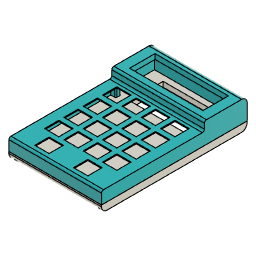
calculator rev1 16122023 (Autodesk Fusion 360 design; units mm, degrees)
Autodesk Fusion 360 part; units mm, degrees
note: some values were not read from the file. Set by a fixed rule: which sketch regions a step uses.
sketch "Sketch1" plane through (0, 0, 0) normal (0, 0, 1) x (1, 0, 0)
  line L0 (-19, 82) -> (72, 82)
  line L1 (72, 82) -> (72, -61)
  line L2 (72, -61) -> (-19, -61)
  line L3 (-19, -61) -> (-19, 82)
  line L4 (-9, 35) -> (5, 35)
  line L5 (5, 35) -> (5, 21)
  line L6 (5, 21) -> (-9, 21)
  line L7 (-9, 21) -> (-9, 35)
  line L8 (10, 35) -> (24, 35)
  line L9 (24, 35) -> (24, 21)
  line L10 (24, 21) -> (10, 21)
  line L11 (10, 21) -> (10, 35)
  line L12 (29, 35) -> (43, 35)
  line L13 (43, 35) -> (43, 21)
  line L14 (43, 21) -> (29, 21)
  line L15 (29, 21) -> (29, 35)
  line L16 (48, 35) -> (62, 35)
  line L17 (62, 35) -> (62, 21)
  line L18 (62, 21) -> (48, 21)
  line L19 (48, 21) -> (48, 35)
  line L20 (-9, 16) -> (5, 16)
  line L21 (5, 16) -> (5, 2)
  line L22 (5, 2) -> (-9, 2)
  line L23 (-9, 2) -> (-9, 16)
  line L24 (10, 16) -> (24, 16)
  line L25 (24, 16) -> (24, 2)
  line L26 (24, 2) -> (10, 2)
  line L27 (10, 2) -> (10, 16)
  line L28 (29, 16) -> (43, 16)
  line L29 (43, 16) -> (43, 2)
  line L30 (43, 2) -> (29, 2)
  line L31 (29, 2) -> (29, 16)
  line L32 (48, 16) -> (62, 16)
  line L33 (62, 16) -> (62, 2)
  line L34 (62, 2) -> (48, 2)
  line L35 (48, 2) -> (48, 16)
  line L36 (-9, -3) -> (5, -3)
  line L37 (5, -3) -> (5, -17)
  line L38 (5, -17) -> (-9, -17)
  line L39 (-9, -17) -> (-9, -3)
  line L40 (10, -3) -> (24, -3)
  line L41 (24, -3) -> (24, -17)
  line L42 (24, -17) -> (10, -17)
  line L43 (10, -17) -> (10, -3)
  line L44 (29, -3) -> (43, -3)
  line L45 (43, -3) -> (43, -17)
  line L46 (43, -17) -> (29, -17)
  line L47 (29, -17) -> (29, -3)
  line L48 (48, -3) -> (62, -3)
  line L49 (62, -3) -> (62, -17)
  line L50 (62, -17) -> (48, -17)
  line L51 (48, -17) -> (48, -3)
  line L52 (-9, -22) -> (5, -22)
  line L53 (5, -22) -> (5, -36)
  line L54 (5, -36) -> (-9, -36)
  line L55 (-9, -36) -> (-9, -22)
  line L56 (10, -22) -> (24, -22)
  line L57 (24, -22) -> (24, -36)
  line L58 (24, -36) -> (10, -36)
  line L59 (10, -36) -> (10, -22)
  line L60 (29, -22) -> (43, -22)
  line L61 (43, -22) -> (43, -36)
  line L62 (43, -36) -> (29, -36)
  line L63 (29, -36) -> (29, -22)
  line L64 (48, -22) -> (62, -22)
  line L65 (62, -22) -> (62, -36)
  line L66 (62, -36) -> (48, -36)
  line L67 (48, -36) -> (48, -22)
  line L68 (0.5, -41) -> (14.5, -41)
  line L69 (14.5, -41) -> (14.5, -55)
  line L70 (14.5, -55) -> (0.5, -55)
  line L71 (0.5, -55) -> (0.5, -41)
  line L72 (38.5, -41) -> (52.5, -41)
  line L73 (52.5, -41) -> (52.5, -55)
  line L74 (52.5, -55) -> (38.5, -55)
  line L75 (38.5, -55) -> (38.5, -41)
  line L76 (-9.5, 73) -> (62.5, 73)
  line L77 (62.5, 73) -> (62.5, 48)
  line L78 (62.5, 48) -> (-9.5, 48)
  line L79 (-9.5, 48) -> (-9.5, 73)
  dimension "d2" = 10
  dimension "d3" = 5
  dimension "d5" = 5
  dimension "d7" = 5
  dimension "d10" = 14
  dimension "d11" = 10
  dimension "d12" = 5
  dimension "d13" = 5
  dimension "d14" = 5
  dimension "d15" = 9.5
  dimension "d16" = 9.5
  dimension "d17" = 14
  dimension "d18" = 5
  dimension "d19" = 5
  dimension "d20" = 25
  dimension "d21" = 72
  dimension "d22" = 91
  dimension "d23" = 9.5
  dimension "d24" = 13
  dimension "d34" = 9
  dimension "d84" = 143
  constraint horizontal L0
  constraint vertical L1
  constraint horizontal L2
  constraint vertical L3
  constraint horizontal L4
  constraint vertical L5
  constraint horizontal L6
  constraint vertical L7
  constraint horizontal L8
  constraint vertical L9
  constraint horizontal L10
  constraint vertical L11
  constraint horizontal L12
  constraint vertical L13
  constraint horizontal L14
  constraint vertical L15
  constraint horizontal L16
  constraint vertical L17
  constraint horizontal L18
  constraint vertical L19
  constraint horizontal L20
  constraint vertical L21
  constraint horizontal L22
  constraint vertical L23
  constraint horizontal L24
  constraint vertical L25
  constraint horizontal L26
  constraint vertical L27
  constraint horizontal L28
  constraint vertical L29
  constraint horizontal L30
  constraint vertical L31
  constraint horizontal L32
  constraint vertical L33
  constraint horizontal L34
  constraint vertical L35
  constraint horizontal L36
  constraint vertical L37
  constraint horizontal L38
  constraint vertical L39
  constraint horizontal L40
  constraint vertical L41
  constraint horizontal L42
  constraint vertical L43
  constraint horizontal L44
  constraint vertical L45
  constraint horizontal L46
  constraint vertical L47
  constraint horizontal L48
  constraint vertical L49
  constraint horizontal L50
  constraint vertical L51
  constraint horizontal L52
  constraint vertical L53
  constraint horizontal L54
  constraint vertical L55
  constraint horizontal L56
  constraint vertical L57
  constraint horizontal L58
  constraint vertical L59
  constraint horizontal L60
  constraint vertical L61
  constraint horizontal L62
  constraint vertical L63
  constraint horizontal L64
  constraint vertical L65
  constraint horizontal L66
  constraint vertical L67
  constraint horizontal L68
  constraint vertical L69
  constraint horizontal L70
  constraint vertical L71
  constraint horizontal L72
  constraint vertical L73
  constraint horizontal L74
  constraint vertical L75
  constraint horizontal L76
  constraint vertical L77
  constraint horizontal L78
  constraint vertical L79
  measures "d2" distance of L3 L7
  measures "d3" distance of L5 L11
  measures "d5" distance of L9 L15
  measures "d7" distance of L13 L19
  measures "d10" distance of L17 L19
  measures "d11" distance of L1 L17
  measures "d12" distance of L6 L20
  measures "d13" distance of L22 L36
  measures "d14" distance of L38 L52
  measures "d15" distance of L57 L69
  measures "d16" distance of L63 L75
  measures "d17" distance of L73 L75
  measures "d18" distance of L58 L68
  measures "d19" distance of L62 L72
  measures "d20" distance of L76 L78
  measures "d21" distance of L77 L79
  measures "d22" distance of L1 L3
  measures "d23" distance of L3 L79
  measures "d24" distance of L4 L78
  measures "d34" distance of L0 L76
  measures "d84" distance of L0 L2
extrude "Extrude1" add sketch "Sketch1" along normal blind 3 makes body 1
sketch "Sketch2" plane through (0, 0, 3) normal (0, 0, 1) x (-1, 0, 0)
  line L0 (-52.5, 55) -> (-38.5, 55)
  line L1 (-38.5, 55) -> (-38.5, 41)
  line L2 (-38.5, 41) -> (-52.5, 41)
  line L3 (-52.5, 41) -> (-52.5, 55)
  line L4 (-62.5, -48) -> (9.5, -48)
  line L5 (9.5, -48) -> (9.5, -73)
  line L6 (9.5, -73) -> (-62.5, -73)
  line L7 (-62.5, -73) -> (-62.5, -48)
  line L8 (-43, -21) -> (-29, -21)
  line L9 (-29, -21) -> (-29, -35)
  line L10 (-29, -35) -> (-43, -35)
  line L11 (-43, -35) -> (-43, -21)
  line L12 (-43, -2) -> (-29, -2)
  line L13 (-29, -2) -> (-29, -16)
  line L14 (-29, -16) -> (-43, -16)
  line L15 (-43, -16) -> (-43, -2)
  line L16 (-24, -2) -> (-10, -2)
  line L17 (-10, -2) -> (-10, -16)
  line L18 (-10, -16) -> (-24, -16)
  line L19 (-24, -16) -> (-24, -2)
  line L20 (-5, -21) -> (9, -21)
  line L21 (9, -21) -> (9, -35)
  line L22 (9, -35) -> (-5, -35)
  line L23 (-5, -35) -> (-5, -21)
  line L24 (-5, -2) -> (9, -2)
  line L25 (9, -2) -> (9, -16)
  line L26 (9, -16) -> (-5, -16)
  line L27 (-5, -16) -> (-5, -2)
  line L28 (-5, 17) -> (9, 17)
  line L29 (9, 17) -> (9, 3)
  line L30 (9, 3) -> (-5, 3)
  line L31 (-5, 3) -> (-5, 17)
  line L32 (-62, -2) -> (-48, -2)
  line L33 (-48, -2) -> (-48, -16)
  line L34 (-48, -16) -> (-62, -16)
  line L35 (-62, -16) -> (-62, -2)
  line L36 (-62, 17) -> (-48, 17)
  line L37 (-48, 17) -> (-48, 3)
  line L38 (-48, 3) -> (-62, 3)
  line L39 (-62, 3) -> (-62, 17)
  line L40 (-43, 17) -> (-29, 17)
  line L41 (-29, 17) -> (-29, 3)
  line L42 (-29, 3) -> (-43, 3)
  line L43 (-43, 3) -> (-43, 17)
  line L44 (-24, 36) -> (-10, 36)
  line L45 (-10, 36) -> (-10, 22)
  line L46 (-10, 22) -> (-24, 22)
  line L47 (-24, 22) -> (-24, 36)
  line L48 (-43, 36) -> (-29, 36)
  line L49 (-29, 36) -> (-29, 22)
  line L50 (-29, 22) -> (-43, 22)
  line L51 (-43, 22) -> (-43, 36)
  line L52 (-62, 36) -> (-48, 36)
  line L53 (-48, 36) -> (-48, 22)
  line L54 (-48, 22) -> (-62, 22)
  line L55 (-62, 22) -> (-62, 36)
  line L56 (-5, 36) -> (9, 36)
  line L57 (9, 36) -> (9, 22)
  line L58 (9, 22) -> (-5, 22)
  line L59 (-5, 22) -> (-5, 36)
  line L60 (-14.5, 55) -> (-0.5, 55)
  line L61 (-0.5, 55) -> (-0.5, 41)
  line L62 (-0.5, 41) -> (-14.5, 41)
  line L63 (-14.5, 41) -> (-14.5, 55)
  line L64 (-24, 17) -> (-10, 17)
  line L65 (-10, 17) -> (-10, 3)
  line L66 (-10, 3) -> (-24, 3)
  line L67 (-24, 3) -> (-24, 17)
  line L68 (-62, -21) -> (-48, -21)
  line L69 (-48, -21) -> (-48, -35)
  line L70 (-48, -35) -> (-62, -35)
  line L71 (-62, -35) -> (-62, -21)
  line L72 (-24, -21) -> (-10, -21)
  line L73 (-10, -21) -> (-10, -35)
  line L74 (-10, -35) -> (-24, -35)
  line L75 (-24, -35) -> (-24, -21)
  line L76 (19, 61) -> (-72, 61)
  line L77 (-72, 61) -> (-72, -82)
  line L78 (-72, -82) -> (19, -82)
  line L79 (19, -82) -> (19, 61)
  line L80 (19, -82) -> (-72, -82)
  line L81 (-72, -82) -> (-72, -43)
  line L82 (-72, -43) -> (19, -43)
  line L83 (19, -43) -> (19, -82)
  dimension "d29" = 5
  constraint horizontal L80
  constraint vertical L81
  constraint horizontal L82
  constraint vertical L83
  constraint coincident L77 L81.end
  constraint coincident L78.end L79.start
  measures "d29" distance of L4 L82
extrude "Extrude2" add sketch "Sketch2" along normal blind 3 contours L77 L78 L79 L80 L81 L82 L83 bodies 1
extrude "Extrude3" add 1 faces at (41.6667, 43, 4) along direction (0, -1, 0) blind 3 on bodies 1 bodies 1
sketch "Sketch3" plane through (0, 0, 0) normal (0, 0, -1) x (1, 0, 0)
  line L0 (-9.5, -48) -> (62.5, -48)
  line L1 (62.5, -48) -> (62.5, -73)
  line L2 (62.5, -73) -> (-9.5, -73)
  line L3 (-9.5, -73) -> (-9.5, -48)
  line L4 (38.5, 55) -> (52.5, 55)
  line L5 (52.5, 55) -> (52.5, 41)
  line L6 (52.5, 41) -> (38.5, 41)
  line L7 (38.5, 41) -> (38.5, 55)
  line L8 (0.5, 55) -> (14.5, 55)
  line L9 (14.5, 55) -> (14.5, 41)
  line L10 (14.5, 41) -> (0.5, 41)
  line L11 (0.5, 41) -> (0.5, 55)
  line L12 (48, 36) -> (62, 36)
  line L13 (62, 36) -> (62, 22)
  line L14 (62, 22) -> (48, 22)
  line L15 (48, 22) -> (48, 36)
  line L16 (29, 36) -> (43, 36)
  line L17 (43, 36) -> (43, 22)
  line L18 (43, 22) -> (29, 22)
  line L19 (29, 22) -> (29, 36)
  line L20 (10, 36) -> (24, 36)
  line L21 (24, 36) -> (24, 22)
  line L22 (24, 22) -> (10, 22)
  line L23 (10, 22) -> (10, 36)
  line L24 (10, 17) -> (24, 17)
  line L25 (24, 17) -> (24, 3)
  line L26 (24, 3) -> (10, 3)
  line L27 (10, 3) -> (10, 17)
  line L28 (29, 17) -> (43, 17)
  line L29 (43, 17) -> (43, 3)
  line L30 (43, 3) -> (29, 3)
  line L31 (29, 3) -> (29, 17)
  line L32 (48, 17) -> (62, 17)
  line L33 (62, 17) -> (62, 3)
  line L34 (62, 3) -> (48, 3)
  line L35 (48, 3) -> (48, 17)
  line L36 (-9, 36) -> (5, 36)
  line L37 (5, 36) -> (5, 22)
  line L38 (5, 22) -> (-9, 22)
  line L39 (-9, 22) -> (-9, 36)
  line L40 (-9, -2) -> (5, -2)
  line L41 (5, -2) -> (5, -16)
  line L42 (5, -16) -> (-9, -16)
  line L43 (-9, -16) -> (-9, -2)
  line L44 (10, -21) -> (24, -21)
  line L45 (24, -21) -> (24, -35)
  line L46 (24, -35) -> (10, -35)
  line L47 (10, -35) -> (10, -21)
  line L48 (29, -21) -> (43, -21)
  line L49 (43, -21) -> (43, -35)
  line L50 (43, -35) -> (29, -35)
  line L51 (29, -35) -> (29, -21)
  line L52 (-9, -21) -> (5, -21)
  line L53 (5, -21) -> (5, -35)
  line L54 (5, -35) -> (-9, -35)
  line L55 (-9, -35) -> (-9, -21)
  line L56 (10, -2) -> (24, -2)
  line L57 (24, -2) -> (24, -16)
  line L58 (24, -16) -> (10, -16)
  line L59 (10, -16) -> (10, -2)
  line L60 (29, -2) -> (43, -2)
  line L61 (43, -2) -> (43, -16)
  line L62 (43, -16) -> (29, -16)
  line L63 (29, -16) -> (29, -2)
  line L64 (48, -2) -> (62, -2)
  line L65 (62, -2) -> (62, -16)
  line L66 (62, -16) -> (48, -16)
  line L67 (48, -16) -> (48, -2)
  line L68 (-9, 17) -> (5, 17)
  line L69 (5, 17) -> (5, 3)
  line L70 (5, 3) -> (-9, 3)
  line L71 (-9, 3) -> (-9, 17)
  line L72 (48, -21) -> (62, -21)
  line L73 (62, -21) -> (62, -35)
  line L74 (62, -35) -> (48, -35)
  line L75 (48, -35) -> (48, -21)
  line L76 (72, 61) -> (-19, 61)
  line L77 (-19, 61) -> (-19, -82)
  line L78 (-19, -82) -> (72, -82)
  line L79 (72, -82) -> (72, 61)
  line L80 (-17, 59) -> (70, 59)
  line L81 (70, 59) -> (70, -80)
  line L82 (70, -80) -> (-17, -80)
  line L83 (-17, -80) -> (-17, 59)
  dimension "d35" = 2
  dimension "d36" = 2
  dimension "d37" = 2
  dimension "d38" = 2
  constraint horizontal L80
  constraint vertical L81
  constraint horizontal L82
  constraint vertical L83
  measures "d35" distance of L79 L81
  measures "d36" distance of L77 L83
  measures "d37" distance of L78 L82
  measures "d38" distance of L76 L80
extrude "Extrude4" cut sketch "Sketch3" against normal blind 2 contours L80 L81 L82 L83 bodies 1
extrude "Extrude5" add 1 faces at (68.8333, 65, 6) along direction (0, 0, 1) blind 10 on bodies 1 bodies 1
sketch "Sketch4" plane through (0, 0, 2) normal (0, 0, -1) x (1, 0, 0)
  line L0 (62, -35) -> (48, -35)
  line L1 (48, -35) -> (48, -21)
  line L2 (48, -21) -> (62, -21)
  line L3 (62, -21) -> (62, -35)
  line L4 (5, 3) -> (-9, 3)
  line L5 (-9, 3) -> (-9, 17)
  line L6 (-9, 17) -> (5, 17)
  line L7 (5, 17) -> (5, 3)
  line L8 (62, -16) -> (48, -16)
  line L9 (48, -16) -> (48, -2)
  line L10 (48, -2) -> (62, -2)
  line L11 (62, -2) -> (62, -16)
  line L12 (43, -16) -> (29, -16)
  line L13 (29, -16) -> (29, -2)
  line L14 (29, -2) -> (43, -2)
  line L15 (43, -2) -> (43, -16)
  line L16 (24, -16) -> (10, -16)
  line L17 (10, -16) -> (10, -2)
  line L18 (10, -2) -> (24, -2)
  line L19 (24, -2) -> (24, -16)
  line L20 (5, -35) -> (-9, -35)
  line L21 (-9, -35) -> (-9, -21)
  line L22 (-9, -21) -> (5, -21)
  line L23 (5, -21) -> (5, -35)
  line L24 (43, -35) -> (29, -35)
  line L25 (29, -35) -> (29, -21)
  line L26 (29, -21) -> (43, -21)
  line L27 (43, -21) -> (43, -35)
  line L28 (24, -35) -> (10, -35)
  line L29 (10, -35) -> (10, -21)
  line L30 (10, -21) -> (24, -21)
  line L31 (24, -21) -> (24, -35)
  line L32 (5, -16) -> (-9, -16)
  line L33 (-9, -16) -> (-9, -2)
  line L34 (-9, -2) -> (5, -2)
  line L35 (5, -2) -> (5, -16)
  line L36 (62.5, -73) -> (-9.5, -73)
  line L37 (-9.5, -73) -> (-9.5, -48)
  line L38 (-9.5, -48) -> (62.5, -48)
  line L39 (62.5, -48) -> (62.5, -73)
  line L40 (24, 3) -> (10, 3)
  line L41 (10, 3) -> (10, 17)
  line L42 (10, 17) -> (24, 17)
  line L43 (24, 17) -> (24, 3)
  line L44 (24, 22) -> (10, 22)
  line L45 (10, 22) -> (10, 36)
  line L46 (10, 36) -> (24, 36)
  line L47 (24, 36) -> (24, 22)
  line L48 (43, 22) -> (29, 22)
  line L49 (29, 22) -> (29, 36)
  line L50 (29, 36) -> (43, 36)
  line L51 (43, 36) -> (43, 22)
  line L52 (62, 22) -> (48, 22)
  line L53 (48, 22) -> (48, 36)
  line L54 (48, 36) -> (62, 36)
  line L55 (62, 36) -> (62, 22)
  line L56 (14.5, 41) -> (0.5, 41)
  line L57 (0.5, 41) -> (0.5, 55)
  line L58 (0.5, 55) -> (14.5, 55)
  line L59 (14.5, 55) -> (14.5, 41)
  line L60 (62, 3) -> (48, 3)
  line L61 (48, 3) -> (48, 17)
  line L62 (48, 17) -> (62, 17)
  line L63 (62, 17) -> (62, 3)
  line L64 (5, 22) -> (-9, 22)
  line L65 (-9, 22) -> (-9, 36)
  line L66 (-9, 36) -> (5, 36)
  line L67 (5, 36) -> (5, 22)
  line L68 (43, 3) -> (29, 3)
  line L69 (29, 3) -> (29, 17)
  line L70 (29, 17) -> (43, 17)
  line L71 (43, 17) -> (43, 3)
  line L72 (52.5, 41) -> (38.5, 41)
  line L73 (38.5, 41) -> (38.5, 55)
  line L74 (38.5, 55) -> (52.5, 55)
  line L75 (52.5, 55) -> (52.5, 41)
  line L76 (-17, -80) -> (70, -80)
  line L77 (70, -80) -> (70, 59)
  line L78 (70, 59) -> (-17, 59)
  line L79 (-17, 59) -> (-17, -80)
  line L80 (70, -80) -> (-17, -80)
  line L81 (-17, -80) -> (-17, -41)
  line L82 (-17, -41) -> (70, -41)
  line L83 (70, -41) -> (70, -80)
  dimension "d43" = 7
  constraint horizontal L80
  constraint vertical L81
  constraint horizontal L82
  constraint vertical L83
  constraint coincident L79 L81.end
  constraint coincident L76.end L77.start
  measures "d43" distance of L38 L82
extrude "Extrude6" cut sketch "Sketch4" against normal blind 9 contours L76 L77 L79 L80 L81 L82 L83 bodies 1
extrude "Extrude7" add 1 faces at (12, 41, 5) along direction (0, 1, 0) blind 1 on bodies 1 bodies 1
extrude "Extrude8" add 1 faces at (71.3333, 33.6667, 0) along direction (0, 0, -1) blind 9 on bodies 1 bodies 1
extrude "Extrude9" cut 1 faces at (68.8333, 65, 16) along direction (0, 0, -1) blind 4 on bodies 1 bodies 1
extrude "Extrude10" add 1 faces at (67.5, 65, 11) along direction (0, 0, -1) blind 4 on bodies 1 bodies 1
fillet "Fillet1" radius 5.5 1 edges at (26.5, 82, 12) on bodies 1
fillet "Fillet2" radius 2 1 edges at (26.5, 40, 12) on bodies 1
fillet "Fillet3" radius 2 1 edges at (26.5, -61, 3) on bodies 1
move_body "Move1" bodies 1 to x (1, 0, 0) y (0, 1, 0) z (0, 0, 1) at (0, 0, 9)
fillet "Fillet4" radius 2 1 edges at (26.5, 40, 12) on bodies 1
move_body "Move2" bodies 1 to x (1, 0, 0) y (0, 1, 0) z (0, 0, 1) at (0, 0, 12)
sketch "Sketch5" plane through (0, 0, 23) normal (0, 0, -1) x (1, 0, 0)
  line L0 (70, -42) -> (70, 59)
  line L1 (70, 59) -> (-17, 59)
  line L2 (-17, 59) -> (-17, -42)
  line L3 (-17, -42) -> (70, -42)
  line L4 (62, -35) -> (48, -35)
  line L5 (48, -35) -> (48, -21)
  line L6 (48, -21) -> (62, -21)
  line L7 (62, -21) -> (62, -35)
  line L8 (5, 3) -> (-9, 3)
  line L9 (-9, 3) -> (-9, 17)
  line L10 (-9, 17) -> (5, 17)
  line L11 (5, 17) -> (5, 3)
  line L12 (62, -16) -> (48, -16)
  line L13 (48, -16) -> (48, -2)
  line L14 (48, -2) -> (62, -2)
  line L15 (62, -2) -> (62, -16)
  line L16 (43, -16) -> (29, -16)
  line L17 (29, -16) -> (29, -2)
  line L18 (29, -2) -> (43, -2)
  line L19 (43, -2) -> (43, -16)
  line L20 (24, -16) -> (10, -16)
  line L21 (10, -16) -> (10, -2)
  line L22 (10, -2) -> (24, -2)
  line L23 (24, -2) -> (24, -16)
  line L24 (5, -35) -> (-9, -35)
  line L25 (-9, -35) -> (-9, -21)
  line L26 (-9, -21) -> (5, -21)
  line L27 (5, -21) -> (5, -35)
  line L28 (43, -35) -> (29, -35)
  line L29 (29, -35) -> (29, -21)
  line L30 (29, -21) -> (43, -21)
  line L31 (43, -21) -> (43, -35)
  line L32 (24, -35) -> (10, -35)
  line L33 (10, -35) -> (10, -21)
  line L34 (10, -21) -> (24, -21)
  line L35 (24, -21) -> (24, -35)
  line L36 (5, -16) -> (-9, -16)
  line L37 (-9, -16) -> (-9, -2)
  line L38 (-9, -2) -> (5, -2)
  line L39 (5, -2) -> (5, -16)
  line L40 (24, 3) -> (10, 3)
  line L41 (10, 3) -> (10, 17)
  line L42 (10, 17) -> (24, 17)
  line L43 (24, 17) -> (24, 3)
  line L44 (24, 22) -> (10, 22)
  line L45 (10, 22) -> (10, 36)
  line L46 (10, 36) -> (24, 36)
  line L47 (24, 36) -> (24, 22)
  line L48 (43, 22) -> (29, 22)
  line L49 (29, 22) -> (29, 36)
  line L50 (29, 36) -> (43, 36)
  line L51 (43, 36) -> (43, 22)
  line L52 (62, 22) -> (48, 22)
  line L53 (48, 22) -> (48, 36)
  line L54 (48, 36) -> (62, 36)
  line L55 (62, 36) -> (62, 22)
  line L56 (14.5, 41) -> (0.5, 41)
  line L57 (0.5, 41) -> (0.5, 55)
  line L58 (0.5, 55) -> (14.5, 55)
  line L59 (14.5, 55) -> (14.5, 41)
  line L60 (62, 3) -> (48, 3)
  line L61 (48, 3) -> (48, 17)
  line L62 (48, 17) -> (62, 17)
  line L63 (62, 17) -> (62, 3)
  line L64 (5, 22) -> (-9, 22)
  line L65 (-9, 22) -> (-9, 36)
  line L66 (-9, 36) -> (5, 36)
  line L67 (5, 36) -> (5, 22)
  line L68 (43, 3) -> (29, 3)
  line L69 (29, 3) -> (29, 17)
  line L70 (29, 17) -> (43, 17)
  line L71 (43, 17) -> (43, 3)
  line L72 (52.5, 41) -> (38.5, 41)
  line L73 (38.5, 41) -> (38.5, 55)
  line L74 (38.5, 55) -> (52.5, 55)
  line L75 (52.5, 55) -> (52.5, 41)
  circle A0 centre (-14.5, -39.5) radius 1.5
  circle A1 centre (67.5, -39.5) radius 1.5
  circle A2 centre (67.5, 56.5) radius 1.5
  circle A3 centre (-14.5, 56.5) radius 1.5
  line L76 (72, 61) -> (-19, 61)
  line L77 (-17, 59) -> (-12, 59)
  line L78 (-12, 59) -> (-12, 54)
  line L79 (-12, 54) -> (-17, 54)
  line L80 (-17, 54) -> (-17, 59)
  line L81 (70, 59) -> (65, 59)
  line L82 (65, 59) -> (65, 54)
  line L83 (65, 54) -> (70, 54)
  line L84 (70, 54) -> (70, 59)
  line L85 (65, -37) -> (70, -37)
  line L86 (70, -37) -> (70, -42)
  line L87 (70, -42) -> (65, -42)
  line L88 (65, -42) -> (65, -37)
  line L89 (-17, -42) -> (-12, -42)
  line L90 (-12, -42) -> (-12, -37)
  line L91 (-12, -37) -> (-17, -37)
  line L92 (-17, -37) -> (-17, -42)
  dimension "d62" = 3
  dimension "d63" = 3
  dimension "d64" = 3
  dimension "d65" = 3
  dimension "d66" = 2.5
  dimension "d67" = 2.5
  dimension "d68" = 2.5
  dimension "d69" = 4.5
  dimension "d70" = 5
  dimension "d71" = 5
  dimension "d72" = 2.5
  dimension "d73" = 2.5
  dimension "d74" = 2.5
  dimension "d75" = 2.5
  dimension "d76" = 5
  dimension "d77" = 5
  dimension "d78" = 5
  dimension "d79" = 5
  constraint horizontal L77
  constraint vertical L78
  constraint horizontal L79
  constraint vertical L80
  constraint coincident L1.end L2.start
  constraint horizontal L81
  constraint vertical L82
  constraint horizontal L83
  constraint vertical L84
  constraint coincident L0.end L1.start
  constraint horizontal L85
  constraint vertical L86
  constraint horizontal L87
  constraint vertical L88
  constraint coincident L0.start L3.end
  constraint horizontal L89
  constraint vertical L90
  constraint horizontal L91
  constraint vertical L92
  constraint coincident L2.end L3.start
  measures "d62" diameter of A0
  measures "d63" diameter of A1
  measures "d64" diameter of A2
  measures "d65" diameter of A3
  measures "d66" distance of L1 A3.centre
  measures "d67" distance of L2 A3.centre
  measures "d68" distance of L0 A2.centre
  measures "d69" distance of A2.centre L76
  measures "d70" distance of L77 L79
  measures "d71" distance of L81 L83
  measures "d72" distance of A0.centre L89
  measures "d73" distance of A0.centre L92
  measures "d74" distance of A1.centre L87
  measures "d75" distance of A1.centre L86
  measures "d76" distance of L85 L87
  measures "d77" distance of L86 L88
  measures "d78" distance of L90 L92
  measures "d79" distance of L89 L91
extrude "Extrude11" add sketch "Sketch5" along normal blind 11 contours L0 L3 L85 L86 L87 L88 | L0 L1 L81 L82 L83 L84 | L2 L3 L89 L90 L91 L92 | L1 L2 L77 L78 L79 L80 bodies 1
fillet "Fillet5" radius 1 6 edges at (65, -54, 17.5) (-12, -54, 17.5) (-12, 42, 17.5) (-12, 37, 17.5) (65, 42, 17.5) (65, 37, 17.5) on bodies 1
move_body "Move3" bodies 1 to x (-1, 0, 0) y (0, 1, 0) z (0, 0, -1) at (144, 0, 54.5153)
sketch "Sketch6" plane through (0, 0, 0) normal (0, 0, 1) x (1, 0, 0)
  line L0 (46, -57.8865) -> (-45, -57.8865)
  line L1 (-45, -57.8865) -> (-45, 85.1135)
  line L2 (-45, 85.1135) -> (46, 85.1135)
  line L3 (46, 85.1135) -> (46, -57.8865)
  dimension "d85" = 143
  dimension "d86" = 91
  constraint horizontal L0
  constraint vertical L1
  constraint horizontal L2
  constraint vertical L3
  measures "d85" distance of L0 L2
  measures "d86" distance of L1 L3
extrude "Extrude12" add sketch "Sketch6" along normal blind 7 separate body makes body 2
fillet "Fillet6" radius 5.5 2 edges at (0.5, -57.8865, 7) (0.5, 85.1135, 7) on bodies 2
sketch "Sketch7" plane through (0, 0, 7) normal (0, 0, 1) x (-1, 0, 0)
  line L0 (-46, -79.6135) -> (45, -79.6135)
  line L1 (45, -79.6135) -> (45, 52.3865)
  line L2 (45, 52.3865) -> (-46, 52.3865)
  line L3 (-46, 52.3865) -> (-46, -79.6135)
  line L4 (28, -77.6135) -> (-30, -77.6135)
  line L5 (-30, -77.6135) -> (-30, -44.6135)
  line L6 (-30, -44.6135) -> (28, -44.6135)
  line L7 (28, -44.6135) -> (28, -77.6135)
  dimension "d91" = 33
  dimension "d92" = 58
  dimension "d93" = 17
  dimension "d94" = 2
  constraint horizontal L4
  constraint vertical L5
  constraint horizontal L6
  constraint vertical L7
  measures "d91" distance of L4 L6
  measures "d92" distance of L5 L7
  measures "d93" distance of L1 L7
  measures "d94" distance of L0 L4
extrude "Extrude13" cut sketch "Sketch7" against normal blind 5 contours L4 L5 L6 L7 bodies 2
extrude "Extrude14" cut 1 faces at (10.6667, 66.6135, 2) along direction (0, 0, -1) blind 2 on bodies 2 bodies 2
sketch "Sketch8" plane through (0, 0, 7) normal (0, 0, 1) x (-1, 0, 0)
  line L0 (-30, -77.6135) -> (-30, -44.6135)
  line L1 (-30, -44.6135) -> (28, -44.6135)
  line L2 (28, -44.6135) -> (28, -77.6135)
  line L3 (28, -77.6135) -> (-30, -77.6135)
  line L4 (-46, -79.6135) -> (45, -79.6135)
  line L5 (45, -79.6135) -> (45, 52.3865)
  line L6 (45, 52.3865) -> (-46, 52.3865)
  line L7 (-46, 52.3865) -> (-46, -79.6135)
  circle A0 centre (40.5, 53.3865) radius 1
  circle A1 centre (-41.5, 53.3865) radius 1
  circle A2 centre (40.5, -42.6135) radius 1
  circle A3 centre (-41.5, -42.6135) radius 1
  line L8 (45, 57.8865) -> (-46, 57.8865)
  dimension "d99" = 2
  dimension "d100" = 2
  dimension "d101" = 2
  dimension "d102" = 2
  dimension "d103" = 4.5
  dimension "d104" = 4.5
  dimension "d105" = 4.5
  dimension "d106" = 4.5
  dimension "d107" = 4.5
  dimension "d108" = 4.5
  dimension "d109" = 100.5
  dimension "d110" = 100.5
  measures "d99" diameter of A0
  measures "d100" diameter of A1
  measures "d101" diameter of A2
  measures "d102" diameter of A3
  measures "d103" distance of A0.centre L8
  measures "d104" distance of L5 A0.centre
  measures "d105" distance of L7 A1.centre
  measures "d106" distance of A1.centre L8
  measures "d107" distance of L7 A3.centre
  measures "d108" distance of L5 A2.centre
  measures "d109" distance of A2.centre L8
  measures "d110" distance of A3.centre L8
extrude "Extrude15" cut sketch "Sketch8" against normal blind 16 contours A1 | A0 | A2 | A3 bodies 2
sketch "Sketch9" plane through (0, 0, 7) normal (0, 0, 1) x (-1, 0, 0)
  circle A0 centre (-41.5, -42.6135) radius 1
  circle A1 centre (40.5, -42.6135) radius 1
  line L0 (-30, -77.6135) -> (-30, -44.6135)
  line L1 (-30, -44.6135) -> (28, -44.6135)
  line L2 (28, -44.6135) -> (28, -77.6135)
  line L3 (28, -77.6135) -> (-30, -77.6135)
  line L4 (-46, -79.6135) -> (45, -79.6135)
  line L5 (45, -79.6135) -> (45, 52.3865)
  line L6 (45, 52.3865) -> (40.5, 52.3865)
  line L7 (40.5, 52.3865) -> (-41.5, 52.3865)
  line L8 (-41.5, 52.3865) -> (-46, 52.3865)
  line L9 (-46, 52.3865) -> (-46, -79.6135)
  circle A2 centre (40.5, -42.6135) radius 2.5
  circle A3 centre (-41.5, -42.6135) radius 2.5
  circle A4 centre (40.5, 53.3865) radius 2.5
  circle A5 centre (-41.5, 53.3865) radius 2.5
  line L10 (45, 57.8865) -> (-46, 57.8865)
  dimension "d113" = 5
  dimension "d114" = 5
  dimension "d115" = 5
  dimension "d116" = 5
  dimension "d117" = 4.5
  dimension "d118" = 4.5
  dimension "d119" = 4.5
  dimension "d120" = 4.5
  constraint concentric A1 A2
  constraint concentric A0 A3
  measures "d113" diameter of A2
  measures "d114" diameter of A3
  measures "d115" diameter of A4
  measures "d116" diameter of A5
  measures "d117" distance of A5.centre L10
  measures "d118" distance of L9 A5.centre
  measures "d119" distance of A4.centre L10
  measures "d120" distance of L5 A4.centre
extrude "Extrude16" cut sketch "Sketch9" against normal blind 2 contours L7 L8 A5 | L7 L8 A5 | L6 L7 A4 | L6 L7 A4 | A2 | A3 bodies 2
copy_body "Body->Comp1" bodies 1 removing the originals makes body 3 in component "main_body"
copy_body "Body->Comp2" bodies 2 removing the originals makes body 4 in component "back"
move_body "Move1'" bodies 4 to x (1, 0, 0) y (0, 1, 0) z (0, 0, 1) at (0, -0.11, 0) in component "back"
fillet "Fillet1'" radius 2 2 edges at (1, 77.5035, 7) (1, 44.5035, 7) on bodies 4 in component "back"
component "main_body" placed x (1, 0, 0) y (0, 1, 0) z (0, 0, 1) at (0, 0, 0)
component "back" placed x (1, 0, 0) y (0, 1, 0) z (0, 0, 1) at (0, 0, 0)
